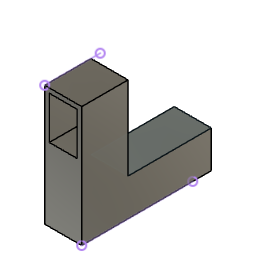
mitad proyecto v1 (Autodesk Fusion 360 design; units mm, degrees)
Autodesk Fusion 360 part; units mm, degrees
sketch "Boceto1" plane through (0, 0, 0) normal (0, 0, 1) x (1, 0, 0)
  line L0 (0, 0) -> (20, 0)
  line L1 (20, 0) -> (20, 30)
  line L2 (20, 30) -> (0, 30)
  line L3 (0, 30) -> (0, 0)
  dimension "d1" = 20
  dimension "d2" = 30
  constraint horizontal L0
  constraint vertical L1
  constraint horizontal L2
  constraint vertical L3
  constraint coincident L0.start L3.end
  measures "d1" distance of L1.end L2.end
  measures "d2" distance of L0.end L1.end
extrude "Extruir1" add sketch "Boceto1" along normal blind 20
extrude "Extruir2" add 1 faces at (13.3333, 30, 6.6667) along direction (0, 1, 0) blind 20
sketch "Boceto2" plane through (0, 0, 0) normal (0, 0, 1) x (1, 0, 0)
  line L0 (20, 0, 20) -> (0, 0, 20)
  line L1 (0, 0, 20) -> (0, 30, 20)
  line L2 (0, 30, 20) -> (20, 30, 20)
  line L3 (20, 30, 20) -> (20, 0, 20)
  dimension "d7" = 30
  dimension "d8" = 20
extrude "Extruir3" add sketch "Boceto2" along normal blind 45 contours L0 L1 L2 L3 in plane through (0, 0, 20) normal (0, 0, 1)
extrude "Extruir4" add 1 faces at (13.3333, 50, 6.6667) along direction (0, 1, 0) blind 10
sketch "Boceto3" plane through (0, 0, 0) normal (0, 0, 1) x (1, 0, 0)
  line L0 (20, 0) -> (20, 60)
  dimension "d13" = 60
  measures "d13" distance of L0.start L0.end
extrude "Extruir5" add 1 faces at (13.3333, 60, 6.6667) along direction (0, 1, 0) blind 10
sketch "Boceto4" plane through (0, 0, 0) normal (0, 0, 1) x (1, 0, 0)
sketch "Boceto5" plane through (0, 0, 0) normal (1, 0, 0) x (0, 1, 0)
  line L0 (0, 65) -> (30, 65)
  dimension "d16" = 30
  measures "d16" distance of L0.start L0.end
extrude "Extruir6" cut 1 faces at (6.6667, 30, 35) along direction (0, -1, 0) blind 5
sketch "Boceto6" plane through (0, 0, 0) normal (0, 1, 0) x (1, 0, 0)
  line L0 (17.5, -62.5) -> (2.5, -62.5)
  line L1 (2.5, -62.5) -> (2.5, -39.5)
  line L2 (2.5, -39.5) -> (17.5, -39.5)
  line L3 (17.5, -39.5) -> (17.5, -62.5)
  dimension "d19" = 15
  dimension "d20" = 23
  constraint horizontal L0
  constraint vertical L1
  constraint horizontal L2
  constraint vertical L3
  measures "d19" distance of L0.start L0.end
  measures "d20" distance of L0.end L1.end
extrude "Extruir7" cut sketch "Boceto6" along normal blind 33
hole "Agujero1" at (9.9694, 25, 63.7746) direction (0, -1, 0) diameter 1 depth 4 tip angle 118
hole "Agujero2" at (10.0421, 25, 38.3) direction (0, -1, 0) diameter 1 depth 4 tip angle 118
sketch "Boceto7" plane through (0, 0, 20) normal (0, 0, 1) x (-1, 0, 0)
  line L0 (-20, -25) -> (-20, -70)
  line L1 (-20, -70) -> (0, -70)
  line L2 (0, -70) -> (0, -25)
  line L3 (0, -25) -> (-20, -25)
sketch "Boceto8" plane through (0, 0, 0) normal (0, 0, 1) x (1, 0, 0)
  line L0 (13.5, 70) -> (6.5, 70)
  line L1 (6.5, 70) -> (6.5, 40)
  line L2 (6.5, 40) -> (13.5, 40)
  line L3 (13.5, 40) -> (13.5, 70)
  dimension "d29" = 30
  dimension "d30" = 7
  constraint horizontal L0
  constraint vertical L1
  constraint horizontal L2
  constraint vertical L3
  measures "d29" distance of L0.start L2.end
  measures "d30" distance of L0.start L0.end
extrude "Extruir8" cut sketch "Boceto8" along normal blind 3
sketch "Boceto9" plane through (0, 0, 0) normal (0, 0, -1) x (1, 0, 0)
  line L0 (13.5, -40) -> (13.5, -70)
  line L1 (13.5, -70) -> (20, -70)
  line L2 (20, -70) -> (20, 0)
  line L3 (20, 0) -> (0, 0)
  line L4 (0, 0) -> (0, -70)
  line L5 (0, -70) -> (6.5, -70)
  line L6 (6.5, -70) -> (6.5, -40)
  line L7 (6.5, -40) -> (13.5, -40)
  line L8 (13.5, -70) -> (12, -70)
  line L9 (12, -70) -> (12, -40)
  line L10 (12, -40) -> (13.5, -40)
  line L11 (13.5, -40) -> (13.5, -70)
  line L12 (6.5, -40) -> (8, -40)
  line L13 (8, -40) -> (8, -70)
  line L14 (8, -70) -> (6.5, -70)
  line L15 (6.5, -70) -> (6.5, -40)
  constraint horizontal L8
  constraint vertical L9
  constraint horizontal L10
  constraint vertical L11
  constraint coincident L7 L9.end
  constraint coincident L0.end L1.start
  constraint horizontal L12
  constraint vertical L13
  constraint horizontal L14
  constraint vertical L15
  constraint coincident L6.end L7.start
extrude "Extruir9" add sketch "Boceto9" against normal blind 1 contours L0 L7 L8 L9 L10 L11
extrude "Extruir10" add 1 faces at (8.8333, 60, 3) along direction (0, 0, -1) blind 1
extrude "Extruir11" cut 1 faces at (8.8333, 60, 2) along direction (0, 0, 1) blind 2
sketch "Boceto10" plane through (0, 0, 0) normal (0, 0, -1) x (1, 0, 0)
  line L0 (12, -70) -> (20, -70)
  line L1 (20, -70) -> (20, 0)
  line L2 (20, 0) -> (0, 0)
  line L3 (0, 0) -> (0, -70)
  line L4 (0, -70) -> (6.5, -70)
  line L5 (6.5, -70) -> (6.5, -40)
  line L6 (6.5, -40) -> (12, -40)
  line L7 (12, -40) -> (12, -70)
  line L8 (6.5, -70) -> (8.1564, -70)
  line L9 (8.1564, -70) -> (8.1564, -40)
  line L10 (8.1564, -40) -> (6.5, -40)
  line L11 (6.5, -40) -> (6.5, -70)
  constraint horizontal L8
  constraint vertical L9
  constraint horizontal L10
  constraint vertical L11
  constraint coincident L6 L9.end
  constraint coincident L4.end L5.start
extrude "Extruir12" add sketch "Boceto10" against normal blind 1 contours L5 L6 L8 L9 L10 L11
